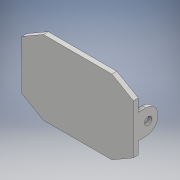
# Autodesk Inventor part: ojo
Saved by Autodesk Inventor 2017 SP1 (Build 210196100, 196)
## iProperties
Part Number: ojo
Material: Genérico
Document SubType Name: Modeling
Designer: Juan
Density: 1 g/cm^3
Appearance: Valor por defecto
Author: Juan
Autodesk Inventor part; units mm, degrees
ref_plane "YZ Plane" through (0, 0, 0) normal (1, 0, 0) x (0, 1, 0)
ref_plane "XZ Plane" through (0, 0, 0) normal (0, 1, 0) x (-1, 0, 0)
ref_plane "XY Plane" through (0, 0, 0) normal (0, 0, 1) x (1, 0, 0)
sketch "Boceto1" plane through (0, 0, 0) normal (0, 1, 0) x (-1, 0, 0)
  line L0 (36.3603, 25) -> (36.3603, 5)
  line L1 (36.3603, 5) -> (27.7, 0)
  line L2 (27.7, 0) -> (0, 0)
  line L3 (0, 0) -> (-8.6603, 5)
  line L4 (-8.6603, 5) -> (-8.6603, 25)
  line L5 (36.3603, 25) -> (27.7, 30.0009)
  line L6 (27.7, 30.0009) -> (0, 30.0009)
  line L7 (0, 30.0009) -> (-8.6603, 25)
  dimension "d0" = 20
  dimension "d1" = 10
  dimension "d2" = 120
  dimension "d3" = 27.7
  dimension "d4" = 150
  dimension "d5" = 10
  dimension "d6" = 150
  dimension "d8" = 27.7
  constraints: 16 end point, 2 vertical, 1 coincident, 1 horizontal, 1 perpendicular
  measures "d0" distance of L0.start L0.end
  measures "d1" distance of L0.end L1.end
  measures "d2" angle of L0 L1
  measures "d3" distance of L1.end L2.end
  measures "d4" angle of L1 L2
  measures "d5" distance of L2.end L3.end
  measures "d6" angle of L2 L3
  measures "d8" distance of L5.end L6.end
extrude "Extrusión1" add sketch "Boceto1" along normal blind 2
sketch "Boceto2" plane through (0, 2, 0) normal (0, 1, 0) x (1, 0, 0)
  line L0 (-27.7, -30.0009) -> (-36.3603, -25) construction
  line L1 (-36.3603, -25) -> (-36.3603, -20) construction
  line L2 (-36.3603, -5) -> (-36.3603, -25) construction
  line L3 (-36.3603, -5) -> (-36.3603, -10) construction
  line L4 (8.6603, -5) -> (8.6603, -25) construction
  line L5 (8.6603, -25) -> (8.6603, -20) construction
  line L6 (8.6603, -5) -> (8.6603, -10) construction
  line L7 (-36.3603, -20) -> (-34.8603, -20)
  line L8 (-34.8603, -20) -> (-34.8603, -10)
  line L9 (-34.8603, -10) -> (-36.3603, -10)
  line L10 (-36.3603, -10) -> (-36.3603, -20)
  line L11 (8.6603, -20) -> (7.1603, -20)
  line L12 (7.1603, -20) -> (7.1603, -10)
  line L13 (7.1603, -10) -> (8.6603, -10)
  line L14 (8.6603, -10) -> (8.6603, -20)
  point P0 (0, 0)
  dimension "d12" = 5
  dimension "d13" = 5
  dimension "d14" = 5
  dimension "d15" = 1.5
  dimension "d16" = 1.5
  constraints: 24 end point, 4 parallel, 3 point on line, 2 horizontal, 2 perpendicular, 1 vertical
  measures "d12" distance of L0.end L1.end
  measures "d13" distance of L2.start L3.end
  measures "d14" distance of L4.end L5.end
  measures "d15" distance of L9.end L8.end
  measures "d16" distance of L12.end L13.end
extrude "Extrusión2" add sketch "Boceto2" along normal blind 8
sketch "Boceto3" plane through (-36.3603, 0, 5) normal (-1, 0, 0) x (0, 0, 1)
  line L0 (15, 10) -> (5, 10) construction
  line L1 (0, 2) -> (5, 2) construction
  line L2 (15, 10) -> (5, 2) construction
  line L3 (10, 6) -> (10, 10) construction
  point P0 (-5, 0)
  constraints: 4 end point, 2 midpoint
hole "Agujero1" at (-36.3603, 6, 15) direction (1, 0, 0) diameter 3 end through all
fillet "Empalme1" radius 5 1 edges at (7.9103, 10, 10)
fillet "Empalme2" radius 5 1 edges at (7.9103, 10, 20)
fillet "Empalme3" radius 5 1 edges at (-35.6103, 10, 10)
fillet "Empalme4" radius 5 1 edges at (-35.6103, 10, 20)
equation "\"d3\" = d8"
